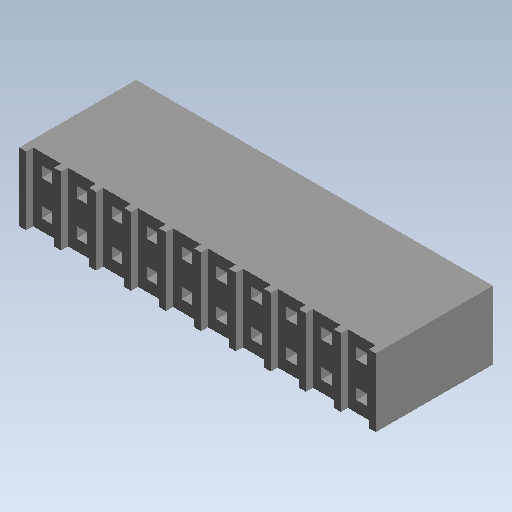
# Autodesk Inventor part: T1SSW-110-02-T-D-RA
Saved by Autodesk Inventor 2021 (Build 250183000, 183)
## iProperties
Part Number: T1SSW-110-02-T-D-RA
Material: Generic
Catalog Web Link: www.cadenas.de
Description: SSW Series Terminal-SSW Series - (2,54 mm) .100" Surface Mount Terminal & Through-Hole .025" Square Post Socket
Vendor: SAMTEC
Document SubType Name: Modeling
Designer: partserver
Manufacturer: SAMTEC
Mass: 0.941555 g
Surface Area: 12.9071 cm^2
Volume: 0.941555 cm^3
Density: 1 g/cm^3
Appearance: PSOLRGB-175-175-175
Category: PARTsolutions
Company: SAMTEC
PSOL_IDENT_0: {$CADENAS_DATA\23d-libs\samtec\modelling\ssw\parts\ssw_terminal.prj},246 {VTYP=3D},{NB=T1SSW-110-02-
PSOL_IDENT_1: T-D-RA},{LINA=T1SSW-110-02-T-D-RA},{NN=SSW Series Terminal},{DATE=08.06.2020 09:25:46},{GEOMDATE=19.
PSOL_IDENT_2: 09.2019 06:31:34},{VERSION=},{LINEID=10},{WBVAR=POS,LS,PLOPT,ROW,TOPT,POLOPT,NOPT,LLOPT,POPT,KOPT,TR
PSOL_IDENT_3: OPT},{WBNUMERIC=}  {NB=T1SSW-110-02-T-D-RA},{LINA=T1SSW-110-02-T-D-RA},{KT=DUMMY},{PN=SSW-110-02-T-D
PSOL_IDENT_4: -RA},{SERIES=SSW},{POS=10},{POSATOF=10},{LS=02},{LSALG= '01','-01','02','-02','03','-03','04','-04','
PSOL_IDENT_5: 06','-06','21','-21','22','-22','23','-23','24','-24' },{PLOPT=T},{PLOPTALG= 'G','-G - Gold, 20micro
PSOL_IDENT_6: \" Au / 50micro\" Ni Min on Contact, 3micro\" Au / 50micro\" Ni Min on Tail','S','-S - Selective, 30
PSOL_IDENT_7: micro\" Au / 50micro\" Ni Min on Contact, Matte Tin Tail','H','-H - Heavy Gold 30micro\" Au / 50micr
PSOL_IDENT_8: o\" Ni Min on Contact, 3micro\" Au / 50micro\" Ni Min on Tail' ,'F','-F - Flash Selective, 3micro\"
PSOL_IDENT_9: Au / 50micro\" Ni Min on Contact, Matte Tin Tail','STL','-STL - Selective, 30micro\" Au / 50micro\"
PSOL_IDENT_10: Ni Min on Contact Area, Tin/Lead (90/10 +/-5%) Tail','SM','-SM - Selective, 30micro\" Au / 50micro\"
PSOL_IDENT_11: Ni Min on Contact, Matte Tin Tail','FM','-FM - Flash Selective, 3micro\" Au / 50micro\" Ni Min on C
PSOL_IDENT_12: ontact, Matte Tin Tail','L','-L - Light Selective, 10micro\" Au / 50micro\" Ni Min on Contact Area,
PSOL_IDENT_13: Matte Tin Tail','T','-T - Matte Tin Contact and Tail','E','-E - 50micro\" Extra Heavy Gold in Contac
PSOL_IDENT_14: t Area, 3micro\" Gold on Tail','TM','-TM - Matte Tin Contact and Tail' },{ROW=D},{ROWALG= 'S','-S -
PSOL_IDENT_15: Single','D','-D - Double','T','-T - Triple', 'P','-P - Single Notched','Q','-Q - Triple with only Ou
PSOL_IDENT_16: ter 2 Rows Filled' },{TOPT=RA},{TOPTALG= '','Straight','RA','-RA - Right Angle' },{TOPTPN=-RA},{POLO
PSOL_IDENT_17: PT=},{POLOPTALG= '','Not Selected','001','001','002','002','003','003','004','004','005','005','006'
PSOL_IDENT_18: ,'006','007','007','008','008','009','009','010','010','011','011','012','012','013','013','014','01
PSOL_IDENT_19: 4','015','015','016','016','017','017','018','018','019','019','020','020' },{POLOPTMAX=240},{POLOPT
PSOL_IDENT_20: MAX2='001','001','002','002','003','003','004','004','005','005','006','006','007','007','008','008'
PSOL_IDENT_21: ,'009','009','010','010','011','011','012','012','013','013','014','014','015','015','016','016','01
PSOL_IDENT_22: 7','017','018','018','019','019','020','020'},{POLARIZE='001','001','002','002','003','003','004','0
PSOL_IDENT_23: 04','005','005','006','006','007','007','008','008','009','009','010','010','011','011','012','012','
PSOL_IDENT_24: 013','013','014','014','015','015','016','016','017','017','018','018','019','019','020','020','021'
PSOL_IDENT_25: ,'021','022','022','023','023','024','024','025','025','026','026','027','027','028','028','029','02
PSOL_IDENT_26: 9','030','030','031','031','032','032','033','033','034','034','035','035','036','036','037','037','
PSOL_IDENT_27: 038','038','039','039','040','040','041','041','042','042','043','043','044','044','045','045','046'
PSOL_IDENT_28: ,'046','047','047','048','048','049','049','050','050','051','051','052','052','053','053','054','05
PSOL_IDENT_29: 4','055','055','056','056','057','057','058','058','059','059','060','060','061','061','062','062','
PSOL_IDENT_30: 063','063','064','064','065','065','066','066','067','067','068','068','069','069','070','070','071'
PSOL_IDENT_31: ,'071','072','072','073','073','074','074','075','075','076','076','077','077','078','078','079','07
PSOL_IDENT_32: 9','080','080','081','081','082','082','083','083','084','084','085','085','086','086','087','087','
PSOL_IDENT_33: 088','088','089','089','090','090','091','091','092','092','093','093','094','094','095','095','096'
PSOL_IDENT_34: ,'096','097','097','098','098','099','099','100','100','101','101','102','102','103','103','104','10
PSOL_IDENT_35: 4','105','105','106','106','107','107','108','108','109','109','110','110','111','111','112','112','
PSOL_IDENT_36: 113','113','114','114','115','115','116','116','117','117','118','118','119','119','120','120','121'
PSOL_IDENT_37: ,'121','122','122','123','123','124','124','125','125','126','126','127','127','128','128','129','12
PSOL_IDENT_38: 9','130','130','131','131','132','132','133','133','134','134','135','135','136','136','137','137','
PSOL_IDENT_39: 138','138','139','139','140','140','141','141','142','142','143','143','144','144','145','145','146'
PSOL_IDENT_40: ,'146','147','147','148','148','149','149','150','150'},{POLOPTPN=},{NOPT=},{NOPTALG= '','Not Select
PSOL_IDENT_41: ed','N','-N - Notch' },{NOPTPN=},{LLOPT=},{LLOPTALG= '','Not Selected','LL','-LL - Locking Lead' },{
PSOL_IDENT_42: LLOPTPN=},{POPT=},{POPTALG= '','Not Available' },{POPTPN=},{KOPT=},{KOPTALG= '','Not Available' },{K
PSOL_IDENT_43: OPTPN=},{TROPT=},{TROPTALG= '','Not Available' },{TROPTPN=},{B=0.194},{C=0.100},{R=1.020},{APOPT=0.3
PSOL_IDENT_44: 1250},{CPOPT=0.39750},{SKOPT=0.38200},{OEN=2},{POSX=0.51500},{POSY=0.01500},{POLOPTATOF=0},{POLMOVE=
PSOL_IDENT_45: 2}
NB: T1SSW-110-02-T-D-RA
NN: SSW Series Terminal
NT: SSW Series - (2,54 mm) .100" Surface Mount Terminal & Through-Hole .025" Square Post Socket
NBSYN: T1$PN.
LINA: T1SSW-110-02-T-D-RA
CATALOG: Samtec
SERIES: SSW
POS: -10
LS: -02
PLOPT: -T - Matte Tin Contact and Tail
ROW: -D - Double
TOPT: -RA - Right Angle
POLOPT: Not Selected
NOPT: Not Selected
LLOPT: Not Selected
POPT: Not Available
KOPT: Not Available
TROPT: Not Available
SUPPLIER: SAMTEC
ARTICLENO: T1SSW-110-02-T-D-RA
BOMINFO: T1SSW-110-02-T-D-RA
CREATOR: CADENAS GmbH
Title: T1SSW-110-02-T-D-RA
Author: Cadenas PARTsolutions
Comments: SSW Series - (2,54 mm) .100" Surface Mount Terminal & Through-Hole .025" Square Post Socket
Autodesk Inventor part; units mm, degrees
sketch "Sketch_1" plane through (0, 0, 0) normal (0, 1, 0) x (-1, 0, 0)
  line L0 (12.954, -2.4765) -> (12.954, 2.4765)
  line L1 (12.954, 2.4765) -> (-12.954, 2.4765)
  line L2 (-12.954, 2.4765) -> (-12.954, -2.4765)
  line L3 (-12.954, -2.4765) -> (12.954, -2.4765)
  line L4 (-11.0363, 0.8763) -> (-11.0363, 1.6637)
  line L5 (-11.0363, 1.6637) -> (-11.8237, 1.6637)
  line L6 (-11.8237, 1.6637) -> (-11.8237, 0.8763)
  line L7 (-11.8237, 0.8763) -> (-11.0363, 0.8763)
  line L8 (-11.0363, -1.6637) -> (-11.0363, -0.8763)
  line L9 (-11.0363, -0.8763) -> (-11.8237, -0.8763)
  line L10 (-11.8237, -0.8763) -> (-11.8237, -1.6637)
  line L11 (-11.8237, -1.6637) -> (-11.0363, -1.6637)
  line L12 (-8.4963, 0.8763) -> (-8.4963, 1.6637)
  line L13 (-8.4963, 1.6637) -> (-9.2837, 1.6637)
  line L14 (-9.2837, 1.6637) -> (-9.2837, 0.8763)
  line L15 (-9.2837, 0.8763) -> (-8.4963, 0.8763)
  line L16 (-8.4963, -1.6637) -> (-8.4963, -0.8763)
  line L17 (-8.4963, -0.8763) -> (-9.2837, -0.8763)
  line L18 (-9.2837, -0.8763) -> (-9.2837, -1.6637)
  line L19 (-9.2837, -1.6637) -> (-8.4963, -1.6637)
  line L20 (-5.9563, 0.8763) -> (-5.9563, 1.6637)
  line L21 (-5.9563, 1.6637) -> (-6.7437, 1.6637)
  line L22 (-6.7437, 1.6637) -> (-6.7437, 0.8763)
  line L23 (-6.7437, 0.8763) -> (-5.9563, 0.8763)
  line L24 (-5.9563, -1.6637) -> (-5.9563, -0.8763)
  line L25 (-5.9563, -0.8763) -> (-6.7437, -0.8763)
  line L26 (-6.7437, -0.8763) -> (-6.7437, -1.6637)
  line L27 (-6.7437, -1.6637) -> (-5.9563, -1.6637)
  line L28 (-3.4163, 0.8763) -> (-3.4163, 1.6637)
  line L29 (-3.4163, 1.6637) -> (-4.2037, 1.6637)
  line L30 (-4.2037, 1.6637) -> (-4.2037, 0.8763)
  line L31 (-4.2037, 0.8763) -> (-3.4163, 0.8763)
  line L32 (-3.4163, -1.6637) -> (-3.4163, -0.8763)
  line L33 (-3.4163, -0.8763) -> (-4.2037, -0.8763)
  line L34 (-4.2037, -0.8763) -> (-4.2037, -1.6637)
  line L35 (-4.2037, -1.6637) -> (-3.4163, -1.6637)
  line L36 (-0.8763, 0.8763) -> (-0.8763, 1.6637)
  line L37 (-0.8763, 1.6637) -> (-1.6637, 1.6637)
  line L38 (-1.6637, 1.6637) -> (-1.6637, 0.8763)
  line L39 (-1.6637, 0.8763) -> (-0.8763, 0.8763)
  line L40 (-0.8763, -1.6637) -> (-0.8763, -0.8763)
  line L41 (-0.8763, -0.8763) -> (-1.6637, -0.8763)
  line L42 (-1.6637, -0.8763) -> (-1.6637, -1.6637)
  line L43 (-1.6637, -1.6637) -> (-0.8763, -1.6637)
  line L44 (1.6637, 0.8763) -> (1.6637, 1.6637)
  line L45 (1.6637, 1.6637) -> (0.8763, 1.6637)
  line L46 (0.8763, 1.6637) -> (0.8763, 0.8763)
  line L47 (0.8763, 0.8763) -> (1.6637, 0.8763)
  line L48 (1.6637, -1.6637) -> (1.6637, -0.8763)
  line L49 (1.6637, -0.8763) -> (0.8763, -0.8763)
  line L50 (0.8763, -0.8763) -> (0.8763, -1.6637)
  line L51 (0.8763, -1.6637) -> (1.6637, -1.6637)
  line L52 (4.2037, 0.8763) -> (4.2037, 1.6637)
  line L53 (4.2037, 1.6637) -> (3.4163, 1.6637)
  line L54 (3.4163, 1.6637) -> (3.4163, 0.8763)
  line L55 (3.4163, 0.8763) -> (4.2037, 0.8763)
  line L56 (4.2037, -1.6637) -> (4.2037, -0.8763)
  line L57 (4.2037, -0.8763) -> (3.4163, -0.8763)
  line L58 (3.4163, -0.8763) -> (3.4163, -1.6637)
  line L59 (3.4163, -1.6637) -> (4.2037, -1.6637)
  line L60 (6.7437, 0.8763) -> (6.7437, 1.6637)
  line L61 (6.7437, 1.6637) -> (5.9563, 1.6637)
  line L62 (5.9563, 1.6637) -> (5.9563, 0.8763)
  line L63 (5.9563, 0.8763) -> (6.7437, 0.8763)
  line L64 (6.7437, -1.6637) -> (6.7437, -0.8763)
  line L65 (6.7437, -0.8763) -> (5.9563, -0.8763)
  line L66 (5.9563, -0.8763) -> (5.9563, -1.6637)
  line L67 (5.9563, -1.6637) -> (6.7437, -1.6637)
  line L68 (9.2837, 0.8763) -> (9.2837, 1.6637)
  line L69 (9.2837, 1.6637) -> (8.4963, 1.6637)
  line L70 (8.4963, 1.6637) -> (8.4963, 0.8763)
  line L71 (8.4963, 0.8763) -> (9.2837, 0.8763)
  line L72 (9.2837, -1.6637) -> (9.2837, -0.8763)
  line L73 (9.2837, -0.8763) -> (8.4963, -0.8763)
  line L74 (8.4963, -0.8763) -> (8.4963, -1.6637)
  line L75 (8.4963, -1.6637) -> (9.2837, -1.6637)
  line L76 (11.8237, 0.8763) -> (11.8237, 1.6637)
  line L77 (11.8237, 1.6637) -> (11.0363, 1.6637)
  line L78 (11.0363, 1.6637) -> (11.0363, 0.8763)
  line L79 (11.0363, 0.8763) -> (11.8237, 0.8763)
  line L80 (11.8237, -1.6637) -> (11.8237, -0.8763)
  line L81 (11.8237, -0.8763) -> (11.0363, -0.8763)
  line L82 (11.0363, -0.8763) -> (11.0363, -1.6637)
  line L83 (11.0363, -1.6637) -> (11.8237, -1.6637)
  constraints: 168 end point
extrude "Extrusion1" add sketch "Sketch_1" along normal blind 8.509
sketch "Sketch_6" plane through (0, 0, 0) normal (0, 0, 1) x (1, 0, 0)
  line L0 (-12.446, -2.032) -> (12.446, -2.032)
  line L1 (12.446, -2.032) -> (12.446, 0.508)
  line L2 (12.446, 0.508) -> (10.414, 0.508)
  line L3 (10.414, 0.508) -> (10.414, -1.27)
  line L4 (10.414, -1.27) -> (9.906, -1.27)
  line L5 (9.906, -1.27) -> (9.906, 0.508)
  line L6 (9.906, 0.508) -> (7.874, 0.508)
  line L7 (7.874, 0.508) -> (7.874, -1.27)
  line L8 (7.874, -1.27) -> (7.366, -1.27)
  line L9 (7.366, -1.27) -> (7.366, 0.508)
  line L10 (7.366, 0.508) -> (5.334, 0.508)
  line L11 (5.334, 0.508) -> (5.334, -1.27)
  line L12 (5.334, -1.27) -> (4.826, -1.27)
  line L13 (4.826, -1.27) -> (4.826, 0.508)
  line L14 (4.826, 0.508) -> (2.794, 0.508)
  line L15 (2.794, 0.508) -> (2.794, -1.27)
  line L16 (2.794, -1.27) -> (2.286, -1.27)
  line L17 (2.286, -1.27) -> (2.286, 0.508)
  line L18 (2.286, 0.508) -> (0.254, 0.508)
  line L19 (0.254, 0.508) -> (0.254, -1.27)
  line L20 (0.254, -1.27) -> (-0.254, -1.27)
  line L21 (-0.254, -1.27) -> (-0.254, 0.508)
  line L22 (-0.254, 0.508) -> (-2.286, 0.508)
  line L23 (-2.286, 0.508) -> (-2.286, -1.27)
  line L24 (-2.286, -1.27) -> (-2.794, -1.27)
  line L25 (-2.794, -1.27) -> (-2.794, 0.508)
  line L26 (-2.794, 0.508) -> (-4.826, 0.508)
  line L27 (-4.826, 0.508) -> (-4.826, -1.27)
  line L28 (-4.826, -1.27) -> (-5.334, -1.27)
  line L29 (-5.334, -1.27) -> (-5.334, 0.508)
  line L30 (-5.334, 0.508) -> (-7.366, 0.508)
  line L31 (-7.366, 0.508) -> (-7.366, -1.27)
  line L32 (-7.366, -1.27) -> (-7.874, -1.27)
  line L33 (-7.874, -1.27) -> (-7.874, 0.508)
  line L34 (-7.874, 0.508) -> (-9.906, 0.508)
  line L35 (-9.906, 0.508) -> (-9.906, -1.27)
  line L36 (-9.906, -1.27) -> (-10.414, -1.27)
  line L37 (-10.414, -1.27) -> (-10.414, 0.508)
  line L38 (-10.414, 0.508) -> (-12.446, 0.508)
  line L39 (-12.446, 0.508) -> (-12.446, -2.032)
  constraints: 80 end point
extrude "Extrusion2" cut sketch "Sketch_6" along normal mid plane 10.16
ref_plane "pin_XY" through (0, 0, 0) normal (0, 1, 0) x (1, 0, 0)
ref_plane "pin_YZ" through (0, 0, 0) normal (1, 0, 0) x (0, 0, -1)
ref_plane "pin_ZX" through (0, 0, 0) normal (0, 0, -1) x (0, 1, 0)
ref_plane "terminal_XY" through (0, 0, 0) normal (0, -1, 0) x (1, 0, 0)
ref_plane "terminal_YZ" through (0, 0, 0) normal (1, 0, 0) x (0, 0, 1)
ref_plane "terminal_ZX" through (0, 0, 0) normal (0, 0, 1) x (0, -1, 0)
body "Solid1"
